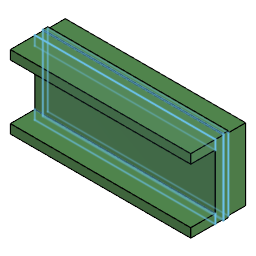
Dhanip_Microcontroller f (Autodesk Fusion 360 design; units mm, degrees)
Autodesk Fusion 360 part; units mm, degrees
note: some values were not read from the file. Set by a fixed rule: which sketch regions a step uses.
sketch "sketch 448" plane through (0, 0, 0) normal (0, 1, 0) x (1, 0, 0)
  line L0 (25.75, -10.75) -> (25.75, 10.75)
  line L1 (25.75, 10.75) -> (-25.75, 10.75)
  line L2 (-25.75, 10.75) -> (-25.75, -10.75)
  line L3 (-25.75, -10.75) -> (25.75, -10.75)
extrude "Extrude1" add sketch "sketch 448" along normal blind 1.4
sketch "sketch 470" plane through (0, 0, 0) normal (0, -1, 0) x (1, 0, 0)
  line L0 (25.75, -10.45) -> (-25.75, -10.45)
  line L1 (25.75, 10.45) -> (25.75, -10.45)
  line L2 (25.75, 10.45) -> (25.75, -10.45)
  line L3 (-25.75, 10.45) -> (25.75, 10.45)
  line L4 (-25.75, -10.45) -> (-25.75, 10.45)
  line L5 (-25.75, -10.45) -> (-25.75, 10.45)
extrude "Extrude2" add sketch "sketch 470" along normal blind 2.3
sketch "sketch 493" plane through (0, -2.3, 0) normal (0, -1, 0) x (1, 0, 0)
  line L0 (25.75, -10.45) -> (-25.75, -10.45)
  line L1 (25.75, -10.45) -> (-25.75, -10.45)
  line L2 (25.75, -7.85) -> (25.75, -10.45)
  line L3 (-25.75, -7.85) -> (25.75, -7.85)
  line L4 (-25.75, -10.45) -> (-25.75, -7.85)
  line L5 (25.75, 7.85) -> (-25.75, 7.85)
  line L6 (25.75, 10.45) -> (25.75, 7.85)
  line L7 (25.75, 10.45) -> (25.75, 7.85)
  line L8 (-25.75, 10.45) -> (25.75, 10.45)
  line L9 (-25.75, 10.45) -> (25.75, 10.45)
  line L10 (-25.75, 7.85) -> (-25.75, 10.45)
  line L11 (-25.75, 7.85) -> (-25.75, 10.45)
extrude "Extrude3" add sketch "sketch 493" along normal blind 7
sketch "sketch 533" plane through (0, 1.4, 0) normal (0, 1, 0) x (-1, 0, 0)
  line L0 (25.75, -10.25) -> (-25.75, -10.25)
  line L1 (25.75, 10.25) -> (25.75, -10.25)
  line L2 (25.75, 10.25) -> (25.75, -10.25)
  line L3 (-25.75, 10.25) -> (25.75, 10.25)
  line L4 (-25.75, -10.25) -> (-25.75, 10.25)
  line L5 (-25.75, -10.25) -> (-25.75, 10.25)
extrude "Extrude4" add sketch "sketch 533" along normal blind 5
